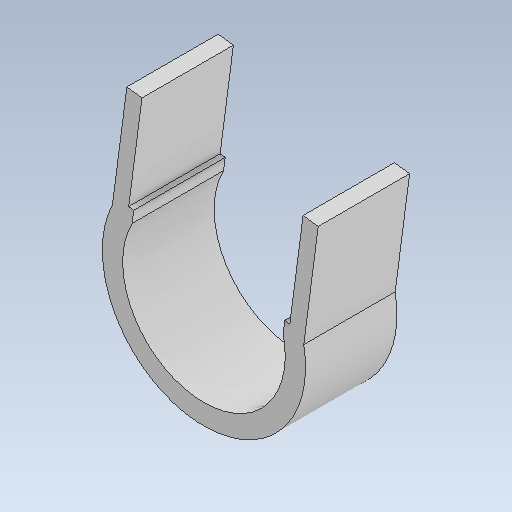
# Autodesk Inventor part: PotHolder
Saved by Autodesk Inventor 2021 (Build 250183000, 183)
## iProperties
Created: 2021-06-05
Part Number: PotHolder
Material: Generic
Document SubType Name: Modeling
Designer: teh18
Density: 1 g/cm^3
Appearance: Default
Author: teh18
Autodesk Inventor part; units mm, degrees
ref_plane "YZ Plane" through (0, 0, 0) normal (1, 0, 0) x (0, 1, 0)
ref_plane "XZ Plane" through (0, 0, 0) normal (0, 1, 0) x (-1, 0, 0)
ref_plane "XY Plane" through (0, 0, 0) normal (0, 0, 1) x (1, 0, 0)
sketch "Sketch1" plane through (0, 0, 0) normal (0, 0, 1) x (1, 0, 0)
  arc A0 (-8.6401, -8.1682) -> (6.2316, -10.1261) centre (-1.5676, -11.9073) ccw
  line L0 (7.4345, -0.9889) -> (6.2316, -10.1261)
  line L1 (-7.4371, 0.969) -> (7.4345, -0.9889)
  line L2 (-8.6401, -8.1682) -> (-7.4371, 0.969)
  line L3 (0.03, -17.852) -> (-0.1568, -19.2714)
  line L4 (-0.1568, -19.2714) -> (-0.6894, -19.2013)
  spline S0 degree 3 poles (-0.6894, -19.2013) (-0.7386, -19.1939) (-0.8276, -19.1805) (-0.9085, -19.1413) (-0.9446, -19.1238) knots 0 0 0 0 0.552879 1 1 1 1
  spline S1 degree 3 poles (-0.9446, -19.1238) (-0.9734, -19.1035) (-1.0308, -19.0631) (-1.0644, -19.0015) (-1.0811, -18.9709) knots 0 0 0 0 0.502328 1 1 1 1
  spline S2 degree 3 poles (-1.0811, -18.9709) (-1.0934, -18.9389) (-1.1175, -18.8762) (-1.1139, -18.8091) (-1.1121, -18.7762) knots 0 0 0 0 0.50999 1 1 1 1
  spline S3 degree 3 poles (-1.1121, -18.7762) (-1.106, -18.7465) (-1.0937, -18.6864) (-1.0581, -18.6365) (-1.0402, -18.6114) knots 0 0 0 0 0.495275 1 1 1 1
  spline S4 degree 3 poles (-1.0402, -18.6114) (-1.0175, -18.5881) (-0.9702, -18.5394) (-0.907, -18.5143) (-0.874, -18.5012) knots 0 0 0 0 0.47813 1 1 1 1
  spline S5 degree 3 poles (-0.874, -18.5012) (-0.912, -18.4819) (-0.9849, -18.4448) (-1.0323, -18.3782) (-1.055, -18.3464) knots 0 0 0 0 0.52153 1 1 1 1
  spline S6 degree 3 poles (-1.055, -18.3464) (-1.071, -18.3116) (-1.1036, -18.2405) (-1.0985, -18.1623) (-1.096, -18.1224) knots 0 0 0 0 0.489114 1 1 1 1
  spline S7 degree 3 poles (-1.096, -18.1224) (-1.09, -18.0901) (-1.0782, -18.0263) (-1.0456, -17.9702) (-1.0294, -17.9425) knots 0 0 0 0 0.505658 1 1 1 1
  spline S8 degree 3 poles (-1.0294, -17.9425) (-1.0117, -17.9179) (-0.9781, -17.8713) (-0.9305, -17.8392) (-0.9079, -17.824) knots 0 0 0 0 0.527149 1 1 1 1
  spline S9 degree 3 poles (-0.9079, -17.824) (-0.8832, -17.8123) (-0.8309, -17.7874) (-0.7736, -17.7788) (-0.7433, -17.7743) knots 0 0 0 0 0.471963 1 1 1 1
  spline S10 degree 3 poles (-0.7433, -17.7743) (-0.7078, -17.7719) (-0.6303, -17.7668) (-0.5531, -17.7758) (-0.5112, -17.7807) knots 0 0 0 0 0.457318 1 1 1 1
  line L5 (-0.5112, -17.7807) -> (0.03, -17.852)
  line L6 (-3.4981, -17.3875) -> (-3.685, -18.8069)
  line L7 (-3.685, -18.8069) -> (-3.8728, -18.7821)
  line L8 (-3.8728, -18.7821) -> (-3.7802, -18.0783)
  line L9 (-3.7802, -18.0783) -> (-4.5777, -18.6893)
  line L10 (-4.5777, -18.6893) -> (-4.8323, -18.6558)
  line L11 (-4.8323, -18.6558) -> (-4.1612, -18.1591)
  line L12 (-4.1612, -18.1591) -> (-4.6716, -17.233)
  line L13 (-4.6716, -17.233) -> (-4.4237, -17.2656)
  line L14 (-4.4237, -17.2656) -> (-4.0129, -18.0506)
  line L15 (-4.0129, -18.0506) -> (-3.7507, -17.8546)
  line L16 (-3.7507, -17.8546) -> (-3.686, -17.3627)
  line L17 (-3.686, -17.3627) -> (-3.4981, -17.3875)
  circle A1 centre (-5.3501, -2.3316) radius 1.25
  circle A2 centre (-0.3929, -2.9842) radius 1.25
  circle A3 centre (4.5643, -3.6369) radius 1.25
  line L18 (-1.8861, -17.5997) -> (-1.7118, -17.6227)
  line L19 (-1.7118, -17.6227) -> (-1.858, -18.7332)
  spline S11 degree 3 poles (-1.858, -18.7332) (-1.8315, -18.7156) (-1.7741, -18.6776) (-1.7111, -18.6498) (-1.6771, -18.6349) knots 0 0 0 0 0.461284 1 1 1 1
  spline S12 degree 3 poles (-1.6771, -18.6349) (-1.6428, -18.6208) (-1.579, -18.5947) (-1.5125, -18.5771) (-1.4818, -18.569) knots 0 0 0 0 0.53896 1 1 1 1
  line L20 (-1.4818, -18.569) -> (-1.5039, -18.7374)
  spline S13 degree 3 poles (-1.5039, -18.7374) (-1.5538, -18.755) (-1.6511, -18.7893) (-1.7387, -18.8438) (-1.7815, -18.8703) knots 0 0 0 0 0.512204 1 1 1 1
  spline S14 degree 3 poles (-1.7815, -18.8703) (-1.8184, -18.8967) (-1.8862, -18.945) (-1.9379, -19.0101) (-1.9614, -19.0397) knots 0 0 0 0 0.545431 1 1 1 1
  line L21 (-1.9614, -19.0397) -> (-2.0737, -19.0249)
  line L22 (-2.0737, -19.0249) -> (-1.8861, -17.5997)
  spline S15 degree 3 poles (-2.4246, -18.241) (-2.4356, -18.317) (-2.4555, -18.4539) (-2.5069, -18.5823) (-2.5297, -18.6393) knots 0 0 0 0 0.555296 1 1 1 1
  spline S16 degree 3 poles (-2.5297, -18.6393) (-2.5543, -18.6843) (-2.6009, -18.7695) (-2.6782, -18.8281) (-2.7148, -18.8558) knots 0 0 0 0 0.527243 1 1 1 1
  spline S17 degree 3 poles (-2.7148, -18.8558) (-2.7553, -18.8752) (-2.84, -18.9157) (-2.9339, -18.9088) (-2.9828, -18.9052) knots 0 0 0 0 0.477983 1 1 1 1
  spline S18 degree 3 poles (-2.9828, -18.9052) (-3.0189, -18.8989) (-3.0882, -18.8866) (-3.1483, -18.8503) (-3.1772, -18.8328) knots 0 0 0 0 0.520451 1 1 1 1
  spline S19 degree 3 poles (-3.1772, -18.8328) (-3.2025, -18.812) (-3.254, -18.7696) (-3.2859, -18.7111) (-3.3021, -18.6815) knots 0 0 0 0 0.49271 1 1 1 1
  spline S20 degree 3 poles (-3.3021, -18.6815) (-3.3159, -18.6476) (-3.3452, -18.5759) (-3.3564, -18.4992) (-3.3624, -18.4588) knots 0 0 0 0 0.472284 1 1 1 1
  spline S21 degree 3 poles (-3.3624, -18.4588) (-3.3653, -18.409) (-3.3719, -18.2955) (-3.358, -18.1825) (-3.3502, -18.1191) knots 0 0 0 0 0.438474 1 1 1 1
  spline S22 degree 3 poles (-3.3502, -18.1191) (-3.3392, -18.0436) (-3.3193, -17.9073) (-3.2684, -17.7795) (-3.2458, -17.7226) knots 0 0 0 0 0.554457 1 1 1 1
  spline S23 degree 3 poles (-3.2458, -17.7226) (-3.2213, -17.6776) (-3.1749, -17.5922) (-3.0976, -17.5334) (-3.0611, -17.5056) knots 0 0 0 0 0.526814 1 1 1 1
  spline S24 degree 3 poles (-3.0611, -17.5056) (-3.0205, -17.4861) (-2.9355, -17.4453) (-2.8413, -17.4522) (-2.792, -17.4558) knots 0 0 0 0 0.477437 1 1 1 1
  spline S25 degree 3 poles (-2.792, -17.4558) (-2.7285, -17.4698) (-2.6047, -17.4969) (-2.5269, -17.5968) (-2.489, -17.6454) knots 0 0 0 0 0.512697 1 1 1 1
  spline S26 degree 3 poles (-2.489, -17.6454) (-2.4583, -17.7269) (-2.386, -17.9186) (-2.4105, -18.1233) (-2.4246, -18.241) knots 0 0 0 0 0.424835 1 1 1 1
  arc A4 (-10.5788, -7.5715) -> (8.2587, -10.0515) centre (-1.5676, -11.9073) ccw
  line L23 (-10.5788, -7.5715) -> (-9.159, 3.213)
  line L24 (-9.159, 3.213) -> (9.6785, 0.733)
  line L25 (9.6785, 0.733) -> (8.2587, -10.0515)
  point P0 (0, 0)
  dimension "d0" = 2
  constraints: 6 end point, 2 point on circle, 1 centre point, 3 other
  measures "d0" distance between parallel lines of L0 L25
ref_plane "Work Plane1" through (-4.5785, -14.9902, 9) normal (0, 0, -1) x (0, 1, 0)
extrude "Extrusion1" add sketch "Sketch1" along normal up to surface (9 mm away) contours L23 L24 L25 A4
sketch "Sketch2" plane through (9.6785, 0.733, 9) normal (0.1305262, 0.9914449, 0) x (0.9914449, -0.1305262, 0)
  line L0 (-17.5, 0) -> (-17.5, 9) projected
  line L1 (-1.5, 0) -> (-1.5, 9) projected
  line L2 (-17.5, 0) -> (-1.5, 0)
  line L3 (-1.5, 0) -> (-1.5, 9)
  line L4 (-1.5, 9) -> (-17.5, 9)
  line L5 (-17.5, 9) -> (-17.5, 0)
  point P0 (-9.5, 9)
  point P1 (-1.5, 0)
  constraints: 8 end point, 2 parallel, 1 horizontal, 1 perpendicular
extrude "Extrusion2" cut sketch "Sketch2" against normal blind 10
body "Solid1"
